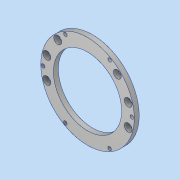
# Autodesk Inventor part: forwardBallastSealingWallDisc
Saved by Autodesk Inventor 2017 (Build 210142000, 142)
## iProperties
Created: 2016-11-26
Part Number: forwardBallastSealingWallDisc
Material: Aluminum 6061
Document SubType Name: Modeling
Designer: techn
Density: 2.7 g/cm^3
Appearance: Aluminum - Flat
Mass: 34.4015 g
Surface Area: 86.6075 cm^2
Volume: 12.7413 cm^3
Author: techn
Autodesk Inventor part; units mm, degrees
ref_plane "YZ Plane" through (0, 0, 0) normal (1, 0, 0) x (0, 1, 0)
ref_plane "XZ Plane" through (0, 0, 0) normal (0, 1, 0) x (-1, 0, 0)
ref_plane "XY Plane" through (0, 0, 0) normal (0, 0, 1) x (1, 0, 0)
sketch "Sketch1" plane through (0, 0, 0) normal (0, 0, 1) x (1, 0, 0)
  circle A0 centre (0, 0) radius 45.212
  line L0 (0, 0) -> (21.4313, 37.12)
  line L1 (0, 0) -> (42.8625, 0) construction
  circle A1 centre (21.4313, 37.12) radius 1.7145
  circle A2 centre (-21.4312, 37.12) radius 1.7145
  circle A3 centre (-42.8625, 0) radius 1.7145
  circle A4 centre (-21.4313, -37.12) radius 1.7145
  circle A5 centre (21.4312, -37.12) radius 1.7145
  circle A6 centre (42.8625, 0) radius 1.7145
  dimension "d0" = 90.424
  dimension "d1" = 42.8625
  dimension "d2" = 60
  dimension "d3" = 3.429
  dimension "d6" = 360
  constraints: 7 centre point, 4 end point, 2 coincident, 1 equal length, 1 horizontal, 13 other
  measures "d0" diameter of A0
  measures "d1" distance of L0.start L0.end
  measures "d2" angle of L1 L0
  measures "d3" diameter of A1
extrude "Extrusion1" add sketch "Sketch1" along normal blind 4.7625
sketch "Sketch2" plane through (0, 0, 4.7625) normal (0, 0, 1) x (1, 0, 0)
  circle A0 centre (0, 0) radius 33.02
  dimension "d10" = 66.04
  constraints: 1 centre point, 1 coincident
  measures "d10" diameter of A0
extrude "Extrusion2" cut sketch "Sketch2" against normal blind 25.4
sketch "Sketch8" plane through (0, 0, 4.7625) normal (0, 0, 1) x (1, 0, 0)
  circle A0 centre (0, 0) radius 33.02 projected
  circle A1 centre (42.8625, 0) radius 1.7145 projected
  circle A2 centre (21.4312, -37.12) radius 1.7145 projected
  circle A3 centre (-21.4313, -37.12) radius 1.7145 projected
  circle A4 centre (-42.8625, 0) radius 1.7145 projected
  circle A5 centre (-21.4312, 37.12) radius 1.7145 projected
  circle A6 centre (21.4313, 37.12) radius 1.7145 projected
  circle A7 centre (0, 0) radius 45.212 projected
  circle A8 centre (0, 0) radius 38.1
  circle A9 centre (39.3779, 10.5513) radius 3.81
  circle A10 centre (39.3779, 10.5513) radius 2.4447
  line L0 (0, 0) -> (39.3779, 10.5513)
  line L1 (0, 0) -> (36.2951, 20.955)
  line L2 (0, 0) -> (41.91, 0) construction
  circle A11 centre (36.2951, 20.955) radius 1.5875
  line L3 (0, 0) -> (0, 9.3613)
  circle A12 centre (39.3779, -10.5513) radius 3.81
  circle A13 centre (-39.3779, 10.5513) radius 3.81
  circle A14 centre (-39.3779, -10.5513) radius 3.81
  circle A15 centre (28.8266, 28.8266) radius 3.81
  line L4 (21.4313, 37.12) -> (0, 0)
  line L5 (0, 0) -> (28.8266, 28.8266)
  circle A16 centre (-28.8266, 28.8266) radius 3.81
  dimension "d37" = 76.2
  dimension "d38" = 7.62
  dimension "d39" = 4.8895
  dimension "d40" = 40.767
  dimension "d42" = 41.91
  dimension "d43" = 30
  dimension "d44" = 3.175
  dimension "d45" = 15
  dimension "d49" = 7.62
  dimension "d50" = 15
  dimension "d51" = 40.767
  constraints: 12 end point, 9 centre point, 4 symmetric about line, 3 coincident, 1 equal length, 1 horizontal, 1 vertical, 4 other
  measures "d37" diameter of A8
  measures "d38" diameter of A9
  measures "d39" diameter of A10
  measures "d40" distance of L0.start L0.end
  measures "d42" distance of L0.start L1.end
  measures "d43" angle of L2 L1
  measures "d44" diameter of A11
  measures "d49" diameter of A15
  measures "d50" angle of L5 L4
  measures "d51" distance of L0.start L5.end
extrude "Extrusion6" cut sketch "Sketch8" against normal blind 25.4 contours L0 A8 A9 | A9 A8 L0 | A9 A8 | A12 A8 | A8 A12 | A13 A8 | A8 A13 | A14 A8 | A8 A14 | A10
extrude "Extrusion7" cut sketch "Sketch8" against normal blind 25.4 contours L5 A8 A15 | A15 A8 L5 | A15 A8 | A16 A8 | A8 A16
equation "\"d49\" = d38"
equation "\"d50\" = d45"
equation "\"d51\" = d40"
body "Solid1"
